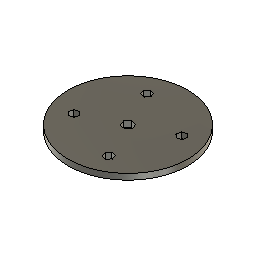
maindisc (Autodesk Fusion 360 design; units mm, degrees)
part number: 2026-05-19-16-48-04-648
Autodesk Fusion 360 part; units mm, degrees
sketch "mainbase" plane through (0, 0, 0) normal (0, 0, 1) x (1, 0, 0)
  circle A0 centre (0, 0) radius 51
  circle A1 centre (0, 0) radius 46.5
  line L0 (-42.0315, -19.8897) -> (5.9278, -46.1206)
  line L1 (5.9278, -46.1206) -> (45.6951, -8.6144)
  line L2 (45.6951, -8.6144) -> (22.3133, 40.7966)
  line L3 (22.3133, 40.7966) -> (-31.9047, 33.8281)
  line L4 (-31.9047, 33.8281) -> (-42.0315, -19.8897)
  line L5 (-31.9047, 33.8281) -> (0, 0)
  line L6 (0, 0) -> (-42.0315, -19.8897)
  line L7 (5.9278, -46.1206) -> (0, 0)
  line L8 (45.6951, -8.6144) -> (0, 0)
  line L9 (22.3133, 40.7966) -> (0, 0)
  line L10 (-20.0354, 17.8663) -> (-16.8802, 20.3249)
  line L11 (-16.8802, 20.3249) -> (-17.4318, 24.2866)
  line L12 (-17.4318, 24.2866) -> (-21.1386, 25.7899)
  line L13 (-21.1386, 25.7899) -> (-24.2938, 23.3313)
  line L14 (-24.2938, 23.3313) -> (-23.7422, 19.3695)
  line L15 (-23.7422, 19.3695) -> (-20.0354, 17.8663)
  line L16 (19.2822, 26.9195) -> (19.1418, 30.9171)
  line L17 (19.1418, 30.9171) -> (15.6096, 32.7942)
  line L18 (15.6096, 32.7942) -> (12.2178, 30.6738)
  line L19 (12.2178, 30.6738) -> (12.3583, 26.6762)
  line L20 (12.3583, 26.6762) -> (15.8905, 24.7991)
  line L21 (15.8905, 24.7991) -> (19.2822, 26.9195)
  line L22 (30.8937, -9.0267) -> (34.6805, -10.315)
  line L23 (34.6805, -10.315) -> (37.6897, -7.6796)
  line L24 (37.6897, -7.6796) -> (36.912, -3.756)
  line L25 (36.912, -3.756) -> (33.1251, -2.4676)
  line L26 (33.1251, -2.4676) -> (30.116, -5.103)
  line L27 (30.116, -5.103) -> (30.8937, -9.0267)
  line L28 (8.3833, -33.8748) -> (6.093, -30.5954)
  line L29 (6.093, -30.5954) -> (2.1078, -30.9391)
  line L30 (2.1078, -30.9391) -> (0.4128, -34.5622)
  line L31 (0.4128, -34.5622) -> (2.7031, -37.8417)
  line L32 (2.7031, -37.8417) -> (6.6883, -37.498)
  line L33 (6.6883, -37.498) -> (8.3833, -33.8748)
  line L34 (-27.3524, -13.6107) -> (-30.2612, -10.865)
  line L35 (-30.2612, -10.865) -> (-34.0934, -12.0112)
  line L36 (-34.0934, -12.0112) -> (-35.0169, -15.9031)
  line L37 (-35.0169, -15.9031) -> (-32.1082, -18.6488)
  line L38 (-32.1082, -18.6488) -> (-28.2759, -17.5026)
  line L39 (-28.2759, -17.5026) -> (-27.3524, -13.6107)
  line L40 (1.4219, -4.5846) -> (4.6813, -1.0609)
  line L41 (4.6813, -1.0609) -> (3.2594, 3.5237)
  line L42 (3.2594, 3.5237) -> (-1.4219, 4.5846)
  line L43 (-1.4219, 4.5846) -> (-4.6813, 1.0609)
  line L44 (-4.6813, 1.0609) -> (-3.2594, -3.5237)
  line L45 (-3.2594, -3.5237) -> (1.4219, -4.5846)
  point P0 (-20.587, 21.8281)
  point P1 (15.75, 28.7966)
  point P2 (33.9028, -6.3913)
  point P3 (4.3981, -34.2185)
  point P4 (-31.1847, -14.7569)
  dimension "d1" = 102
  dimension "d2" = 93
  dimension "d3" = 46.5
  dimension "d4" = 4
  dimension "d5" = 12
  dimension "d6" = 4
  dimension "d7" = 12
  dimension "d8" = 4
  dimension "d9" = 12
  dimension "d10" = 4
  dimension "d11" = 12
  dimension "d12" = 4
  dimension "d13" = 12
  dimension "d14" = 4.8
  constraint coincident A0.centre A1.centre
  constraint concentric A0 A1
  constraint coincident L5 P0
  constraint coincident L9 P1
  constraint coincident L8 P2
  constraint coincident L7 P3
  constraint coincident L6 P4
  measures "d1" diameter of A0
  measures "d2" diameter of A1
  measures "d3" distance of L0.start A0.centre
  measures "d4" distance of L10.start P0
  measures "d5" vertical distance of L3.end P0
  measures "d6" distance of L16.start P1
  measures "d7" vertical distance of L2.end P1
  measures "d8" distance of L22.start P2
  measures "d9" distance of L1.end P2
  measures "d10" distance of L28.start P3
  measures "d11" distance of L0.end P3
  measures "d12" distance of L34.start P4
  measures "d13" distance of L0.start P4
  measures "d14" distance of L40.start A0.centre
extrude "Extrude1" add sketch "mainbase" along normal blind 5 contours A0 | A1 L2 | A1 L3 | L3 L5 L9 L10 L11 L12 L13 L17 L18 L19 L20 L42 L43 | L2 L8 L9 L16 L17 L20 L21 L24 L25 L26 L27 L41 L42 | A1 L1 | L1 L7 L8 L22 L23 L24 L27 L28 L29 L32 L33 L40 L41 L45 | A1 L4 | L4 L5 L6 L10 L13 L14 L15 L34 L35 L36 L37 L43 L44 | L9 L16 L17 L20 L21 | L9 L17 L18 L19 L20 | A1 L0 | L0 L6 L7 L29 L30 L31 L32 L34 L37 L38 L39 L44 L45 | L8 L22 L23 L24 L27 | L8 L24 L25 L26 L27 | L5 L10 L11 L12 L13 | L5 L10 L13 L14 L15 | L7 L29 L30 L31 L32 | L7 L28 L29 L32 L33 | L6 L34 L35 L36 L37 | L6 L34 L37 L38 L39
extrude "Extrude2" cut sketch "mainbase" along normal blind 25 contours L6 L34 L35 L36 L37 | L6 L34 L37 L38 L39
pattern_circular "C-Pattern1" count 4 over 360 about axis through (0, 0, 1.75) along (0, 0, 1) of "Extrude2"
equation "d3 = ( 93 / 2 ) * 1 mm"
named bodies: "maindisc"
